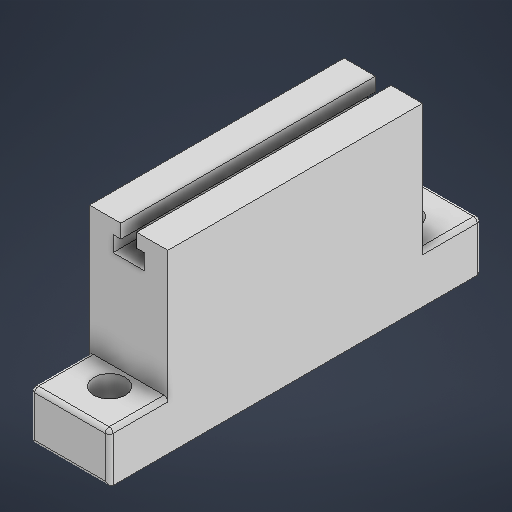
# Autodesk Inventor part: Support
Saved by Autodesk Inventor 2026.2 (Build 302298010, 298A)
## iProperties
Created: 2026-04-28
Part Number: Support
Material: Générique
Document SubType Name: Modeling
Designer: romai
Density: 1 g/cm^3
Appearance: Par défaut
Author: romai
Autodesk Inventor part; units mm, degrees
ref_plane "YZ Plane" through (0, 0, 0) normal (1, 0, 0) x (0, 1, 0)
ref_plane "XZ Plane" through (0, 0, 0) normal (0, 1, 0) x (-1, 0, 0)
ref_plane "XY Plane" through (0, 0, 0) normal (0, 0, 1) x (1, 0, 0)
sketch "Esquisse1" plane through (0, 0, 0) normal (0, 1, 0) x (-1, 0, 0)
  line L0 (-20, 65) -> (20, 65)
  line L1 (20, 65) -> (20, -65)
  line L2 (20, -65) -> (-20, -65)
  line L3 (-20, -65) -> (-20, 65)
  line L4 (-20, 65) -> (20, -65) construction
  line L5 (20, 65) -> (-20, -65) construction
  point P0 (0, 0)
  dimension "d0" = 40
  dimension "d1" = 130
  constraints: 12 end point, 2 midpoint, 2 parallel, 1 horizontal, 1 perpendicular
  measures "d0" distance of L1.end L2.end
  measures "d1" distance of L0.end L1.end
extrude "Extrusion1" add sketch "Esquisse1" along normal mid plane 90
sketch "Esquisse2" plane through (20, 45, -65) normal (0, 0, -1) x (-1, 0, 0)
  line L0 (0, 0) -> (40, 0) projected
  line L1 (16, 0) -> (16, -7)
  line L2 (16, -7) -> (12, -7)
  line L3 (12, -7) -> (12, -15)
  line L4 (20, 0.6313) -> (20, -19.069)
  line L5 (12, -15) -> (20, -15)
  line L6 (24, 0) -> (24, -7)
  line L7 (24, -7) -> (28, -7)
  line L8 (28, -7) -> (28, -15)
  line L9 (28, -15) -> (20, -15)
  point P0 (20, -45)
  point P1 (20, 0)
  dimension "d4" = 7
  dimension "d5" = 4
  dimension "d6" = 4
  dimension "d7" = 8
  constraints: 18 end point, 4 symmetric about line, 3 perpendicular, 2 point on line, 1 horizontal, 1 midpoint, 1 vertical
  measures "d4" distance of L1.start L1.end
  measures "d5" distance from line of point (20, 0) L1
  measures "d6" distance of L1.end L2.end
  measures "d7" distance of L2.end L3.end
extrude "Extrusion2" cut sketch "Esquisse2" against normal through all
sketch "Esquisse3" plane through (-20, -45, 65) normal (0, 0, 1) x (1, 0, 0)
  line L0 (40, 0) -> (40, 90) projected
  line L1 (0, 25) -> (40, 25)
  line L2 (40, 25) -> (40, 0)
  line L3 (40, 0) -> (0, 0)
  line L4 (0, 0) -> (0, 25)
  line L5 (0, 25) -> (40, 0) construction
  line L6 (40, 25) -> (0, 0) construction
  point P0 (20, 45)
  point P1 (20, 12.5)
  dimension "d10" = 25
  constraints: 12 end point, 2 midpoint, 2 parallel, 1 horizontal, 1 perpendicular
  measures "d10" distance of L3.end L1.start
extrude "Extrusion3" add sketch "Esquisse3" along normal blind 30
fillet "Congé1" radius 2 6 edges at (20, -20, 80) (20, -32.5, 95) (0, -20, 95) (-20, -20, 80) (-20, -32.5, 95) (0, -45, 95)
sketch "Esquisse4" plane through (-18, -20, 65) normal (0, 1, 0) x (1, 0, 0)
  line L0 (0, -28) -> (0, 0) projected
  line L1 (36, -28) -> (0, -28) projected
  line L2 (36, 0) -> (36, -28) projected
  line L3 (0, 0) -> (36, 0) projected
  line L4 (46, 65) -> (-10, 65) projected
  point P0 (18, 65)
  point P1 (18.2732, -10)
  dimension "d21" = 75
  measures "d21" distance from line of point (18.273, -10) L4
hole "Perçage1" at (0.2732, -20, 75) direction (0, -1, 0) diameter 16 end through all
mirror "Mise en miroir2" about plane through (0, 0, 0) normal (0, 0, 1) of "Extrusion3", "Congé1", "Perçage1"
